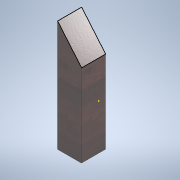
# Autodesk Inventor part: NestArmP2-ver1-1111-2021
Saved by Autodesk Inventor 2021 (Build 250183000, 183)
## iProperties
Created: 2021-03-02
Part Number: NestArmP2-ver1-1111-2021
Material: Generic
Document SubType Name: Modeling
Designer: CMurray
Density: 1 g/cm^3
Appearance: Wild Cherry - Wild Berries
Author: CMurray
Autodesk Inventor part; units mm, degrees
ref_plane "YZ Plane" through (0, 0, 0) normal (1, 0, 0) x (0, 1, 0)
ref_plane "XZ Plane" through (0, 0, 0) normal (0, 1, 0) x (-1, 0, 0)
ref_plane "XY Plane" through (0, 0, 0) normal (0, 0, 1) x (1, 0, 0)
sketch "Sketch1" plane through (0, 0, 0) normal (0, 1, 0) x (-1, 0, 0)
  line L0 (0, 0) -> (127, 0)
  line L1 (127, 0) -> (127, -127)
  line L2 (127, -127) -> (0, -127)
  line L3 (0, -127) -> (0, 0)
  dimension "d0" = 127
  dimension "d1" = 127
  constraints: 8 end point, 2 parallel, 1 horizontal, 1 perpendicular
  measures "d0" distance between parallel lines of L2 L0
  measures "d1" distance between parallel lines of L3 L1
extrude "Extrusion1" add sketch "Sketch1" along normal blind 254
sketch "Sketch2" plane through (0, 254, 0) normal (0, 1, 0) x (1, 0, 0)
  line L0 (-127, 0) -> (0, 0) projected
  line L1 (-127, 127) -> (-127, 0) projected
  line L2 (0, 0) -> (-127, 0)
  line L3 (-127, 0) -> (-127, 127)
  line L4 (-127, 127) -> (0, 127)
  line L5 (0, 127) -> (0, 0)
  constraints: 8 end point, 2 parallel, 1 horizontal, 1 perpendicular
extrude "Extrusion2" add sketch "Sketch2" along normal blind 127
ref_plane "Work Plane1" through (0, 381, 0) normal (-0.7660444, -0.6427876, 0) x (0, 0, -1)
sketch "Sketch4" plane through (0, 381, 0) normal (-0.7660444, -0.6427876, 0) x (0, 0, -1)
  line L0 (-9.5876, -147.9681) -> (139.0202, -147.9681)
  line L1 (139.0202, -147.9681) -> (139.0202, 162.4304)
  line L2 (139.0202, 162.4304) -> (-9.5876, 162.4304)
  line L3 (-9.5876, 162.4304) -> (-9.5876, -147.9681)
  point P0 (0, 291.8629)
  constraints: 8 end point, 2 parallel, 1 horizontal, 1 perpendicular
extrude "Extrusion3" cut sketch "Sketch4" along normal blind 127
sketch "Sketch5" plane through (0, 0, 0) normal (0, -1, 0) x (1, 0, 0)
  line L0 (-127, 0) -> (0, 0) projected
  line L1 (-127, -127) -> (-127, 0) projected
  line L2 (0, 0) -> (-127, 0)
  line L3 (-127, 0) -> (-127, -127)
  line L4 (-127, -127) -> (0, -127)
  line L5 (0, -127) -> (0, 0)
  constraints: 8 end point, 2 parallel, 1 horizontal, 1 perpendicular
extrude "Extrusion4" add sketch "Sketch5" along normal blind 254
sketch "Sketch6" plane through (-97.2876, 299.366, 0) normal (0.7660444, 0.6427876, 0) x (0, 0, -1)
  line L0 (127, -151.3527) -> (0, -151.3527) projected
  line L1 (0, 46.2242) -> (127, 46.2242) projected
  line L2 (0, -151.3527) -> (127, -151.3527)
  line L3 (127, -151.3527) -> (127, 46.2242)
  line L4 (127, 46.2242) -> (0, 46.2242)
  line L5 (0, 46.2242) -> (0, -151.3527)
  point P0 (0, -291.8629)
  constraints: 8 end point, 2 parallel, 1 horizontal, 1 perpendicular
body "Solid1"
